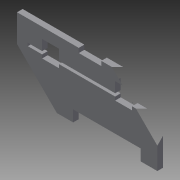
# Autodesk Inventor part: RearBulkhead
Saved by Autodesk Inventor 2014 (Build 180170000, 170)
## iProperties
Created: 2015-01-07
Part Number: RearBulkhead
Material: Generic
Document SubType Name: Modeling
Designer: Owner
Density: 1 g/cm^3
Appearance: Default
Author: Owner
Autodesk Inventor part; units mm, degrees
ref_plane "YZ Plane" through (0, 0, 0) normal (1, 0, 0) x (0, 1, 0)
ref_plane "XZ Plane" through (0, 0, 0) normal (0, 1, 0) x (-1, 0, 0)
ref_plane "XY Plane" through (0, 0, 0) normal (0, 0, 1) x (1, 0, 0)
sketch "Sketch1" plane through (0, 0, 0) normal (0, 0, 1) x (1, 0, 0)
  line L0 (60.3753, 90.1264) -> (-18.9997, 90.1264)
  line L1 (-18.9997, 90.1264) -> (-18.9997, 52.0264)
  line L2 (-18.9997, 52.0264) -> (60.3753, 52.0264)
  line L3 (60.3753, 52.0264) -> (60.3753, 90.1264)
  line L4 (60.3753, 78.1884) -> (-18.9997, 78.1884)
  line L5 (-18.9997, 78.1884) -> (-18.9997, 76.5584)
  line L6 (-18.9997, 76.5584) -> (60.3753, 76.5584)
  line L7 (60.3753, 76.5584) -> (60.3753, 78.1884)
  line L8 (54.4063, 78.1884) -> (54.4063, 76.5584)
  line L9 (-12.9037, 76.5584) -> (-12.9037, 78.1884)
  point P0 (0, 0)
  dimension "d0" = 38.1
  dimension "d1" = 79.375
  dimension "d2" = 1.63
  dimension "d3" = 11.938
  dimension "d6" = 67.31
  dimension "d7" = 6.096
  constraints: 20 end point, 6 point on line, 4 parallel, 4 perpendicular, 2 horizontal
  measures "d0" distance of L0.end L1.end
  measures "d1" distance of L0.start L0.end
  measures "d2" distance between parallel lines of L6 L4
  measures "d3" distance between parallel lines of L0 L4
  measures "d6" distance between parallel lines of L8 L9
  measures "d7" distance between parallel lines of L1 L9
extrude "Extrusion1" add sketch "Sketch1" along normal blind 3.175 contours L3 L4 L1 L0 | L3 L6 L8 L4 | L4 L9 L6 L1 | L3 L2 L1 L6
sketch "Sketch2" plane through (0, 0, 0) normal (0, 0, -1) x (-1, 0, 0)
  line L0 (-54.4063, 78.1884) -> (12.9037, 78.1884) projected
  line L1 (12.9037, 78.1884) -> (12.9037, 76.5584) projected
  line L2 (-4.7145, 84.1043) -> (4.8105, 84.1043)
  line L3 (4.8105, 84.1043) -> (4.8105, 74.5793)
  line L4 (4.8105, 74.5793) -> (-4.7145, 74.5793)
  line L5 (-4.7145, 74.5793) -> (-4.7145, 84.1043)
  line L6 (-46.009, 84.1043) -> (-36.484, 84.1043)
  line L7 (-36.484, 84.1043) -> (-36.484, 74.5865)
  line L8 (-36.484, 74.5865) -> (-46.009, 74.5865)
  line L9 (-46.009, 74.5865) -> (-46.009, 84.1043)
  line L10 (18.9997, 52.0264) -> (-60.3753, 52.0264) projected
  line L11 (18.9997, 90.1264) -> (18.9997, 52.0264) projected
  line L12 (-50.8503, 52.0264) -> (-12.7503, 52.0264)
  line L13 (-12.7503, 52.0264) -> (-12.7503, 58.3764)
  line L14 (-12.7503, 58.3764) -> (-50.8503, 58.3764)
  line L15 (-50.8503, 58.3764) -> (-50.8503, 52.0264)
  line L16 (-60.3753, 52.0264) -> (-60.3753, 90.1264) projected
  line L17 (-60.3753, 90.1264) -> (18.9997, 90.1264) projected
  line L18 (-28.6253, 90.1264) -> (-15.9253, 90.1264)
  line L19 (-15.9253, 90.1264) -> (-15.9253, 87.5864)
  line L20 (-15.9253, 87.5864) -> (-28.6253, 87.5864)
  line L21 (-28.6253, 87.5864) -> (-28.6253, 90.1264)
  point P0 (0, 0)
  dimension "d8" = 9.525
  dimension "d9" = 9.5177
  dimension "d10" = 9.525
  dimension "d11" = 9.525
  dimension "d12" = 31.7695
  dimension "d13" = 5.9159
  dimension "d14" = 8.0932
  dimension "d17" = 6.35
  dimension "d18" = 38.1
  dimension "d19" = 31.75
  dimension "d20" = 2.54
  dimension "d21" = 12.7
  dimension "d22" = 31.75
  constraints: 32 end point, 8 parallel, 4 horizontal, 4 perpendicular, 2 point on line
  measures "d8" distance of L6.start L6.end
  measures "d9" distance of L6.end L7.end
  measures "d10" distance of L2.start L2.end
  measures "d11" distance of L4.end L2.start
  measures "d12" distance between parallel lines of L5 L7
  measures "d13" distance between parallel lines of L0 L2
  measures "d14" distance between parallel lines of L1 L3
  measures "d17" distance of L12.end L13.end
  measures "d18" distance of L13.end L14.end
  measures "d19" distance between parallel lines of L11 L13
  measures "d20" distance of L18.end L19.end
  measures "d21" distance of L19.end L20.end
  measures "d22" distance between parallel lines of L16 L21
extrude "Extrusion2" cut sketch "Sketch2" against normal blind 3.175 contours L9 L6 L7 L0 | L0 L7 L8 L9 | L5 L2 L3 L0 | L0 L3 L4 L5 | L10 L15 L14 L13 | L19 L20 L21 L17
body "Solid1"
